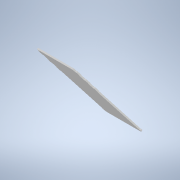
# Autodesk Inventor part: Rampa
Saved by Autodesk Inventor 2020.1 (Build 241239000, 239)
## iProperties
Created: 2019-12-08
Part Number: Rampa
Material: Generic
Document SubType Name: Modeling
Designer: Daniel
Density: 1 g/cm^3
Appearance: Default
Author: Daniel
Autodesk Inventor part; units mm, degrees
ref_plane "YZ Plane" through (0, 0, 0) normal (1, 0, 0) x (0, 1, 0)
ref_plane "XZ Plane" through (0, 0, 0) normal (0, 1, 0) x (-1, 0, 0)
sketch "Sketch2" plane through (0, 0, 0) normal (1, 0, 0) x (0, 1, 0)
  line L0 (-114, -127.2132) -> (-112.153, -129.5772)
  line L1 (-112.153, -129.5772) -> (84, 23.6743)
  line L2 (-114, -127.2132) -> (-114, -57.4172)
  line L3 (-114, -57.4172) -> (-84, -33.9786)
  circle A0 centre (0, 5) radius 17.5
  circle A1 centre (0, 5) radius 31
  line L4 (-114, -127.2132) -> (84, 27.4814)
  line L5 (84, -40) -> (84, 40)
  line L6 (-84, -40) -> (84, -40)
  line L7 (76.1199, 17.5177) -> (74.2729, 19.8817)
  line L8 (64.2997, 8.2828) -> (62.4527, 10.6468)
  line L9 (-84, 40) -> (-84, -40)
  line L10 (84, 40) -> (-84, 40)
  line L11 (38.2954, -12.034) -> (36.4484, -9.67)
  line L12 (50.1155, -2.7991) -> (48.2686, -0.4351)
  line L13 (12.291, -32.3509) -> (10.444, -29.9868)
  line L14 (24.1112, -23.116) -> (22.2642, -20.7519)
  line L15 (83.212, 23.0587) -> (81.365, 25.4227)
  point P0 (0, 0)
  dimension "d49" = 3
  dimension "d37" = 62
  dimension "d38" = 35
  dimension "d39" = 142
  dimension "d40" = 168
  dimension "d41" = 198
  dimension "d42" = 15
  dimension "d43" = 33
  dimension "d44" = 48
  dimension "d45" = 66
  dimension "d46" = 81
  dimension "d47" = 238.9218
  dimension "d48" = 80
  dimension "d50" = 58
  dimension "d51" = 84
  dimension "d52" = 70.7683
  dimension "d53" = 40
  dimension "d54" = 84
  dimension "d55" = 67.69
  dimension "d56" = 1
  constraints: 28 end point, 8 parallel, 3 perpendicular, 3 point on line, 2 centre point, 1 vertical, 24 other
  measures "d37" diameter of A1
  measures "d38" diameter of A0
  measures "d39" angle of L7 L5
  measures "d40" distance between parallel lines of L9 L5
  measures "d41" distance between parallel lines of L2 L5
  measures "d42" distance between parallel lines of L7 L8
  measures "d43" distance between parallel lines of L7 L12
  measures "d44" distance between parallel lines of L7 L11
  measures "d45" distance between parallel lines of L7 L14
  measures "d46" distance between parallel lines of L7 L13
  measures "d47" distance between parallel lines of L7 L0
  measures "d48" distance between parallel lines of L10 L6
  measures "d51" distance from line of point (0, 0) L5
  measures "d52" distance from line of point (0, 0) L7
  measures "d53" distance from line of point (0, 0) L10
  measures "d54" distance from line of A0.centre L5
  measures "d55" distance from line of A0.centre L7
  measures "d56" distance from line of point (84, 23.674) L15
extrude "Extrusion1" add sketch "Sketch2" along normal blind 82 contours L4 L6 L1 L0 | L4 L13 L1 L6 | L4 L14 L1 L13 | L4 L11 L1 L14 | L4 L12 L1 L11 | L1 L7 L4 L15 | L4 L8 L1 L12 | L1 L8 L4 L7
extrude "Extrusion2" add sketch "Sketch2" against normal blind 3 contours L4 L14 L1 L13 | L4 L12 L1 L11 | L1 L8 L4 L7
ref_plane "Work Plane1" through (41, 0, 0) normal (-1, 0, 0) x (0, 0, 1)
mirror "Mirror1" about plane through (41, 0, 0) normal (-1, 0, 0) of "Extrusion2"
sketch "Sketch3" plane through (82, 34.1157, -15.2995) normal (0, 0.6156615, -0.7880108) x (-1, 0, 0)
  line L0 (-3, -195.6177) -> (85, -195.6177)
  line L1 (-3, -185.6177) -> (-3, -195.6177)
  line L2 (85, -185.6177) -> (85, -195.6177)
  line L3 (82, -185.6177) -> (82, -27.696) projected
  line L4 (0, -185.6177) -> (0, -27.696) projected
  line L5 (82, -185.6177) -> (0, -185.6177) projected
  line L6 (-3, -185.6177) -> (85, -185.6177)
  dimension "d57" = 10
  dimension "d58" = 3
  dimension "d59" = 3
  constraints: 8 end point, 1 collinear, 1 horizontal, 1 parallel, 1 vertical
  measures "d57" distance between parallel lines of L0 L6
  measures "d58" distance between parallel lines of L3 L2
  measures "d59" distance between parallel lines of L4 L1
extrude "Extrusion3" add sketch "Sketch3" against normal up to surface (3 mm away)
fillet "Fillet1" radius 10 2 edges at (85, -120.9566, -134.5518) (-3, -120.9566, -134.5518)
body "Solid1"
